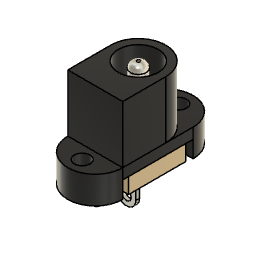
Con_DC-13B_PJ-038BH (Autodesk Fusion 360 design; units mm, degrees)
Autodesk Fusion 360 part; units mm, degrees
note: some values were not read from the file. Set by a fixed rule: which sketch regions a step uses.
sketch "Sketch11" plane through (0, 0, 0) normal (0, 0, 1) x (1, 0, 0)
  circle A0 centre (0, 0) radius 1.25
  circle A1 centre (0, 0) radius 3.2
  line L0 (-10, 0) -> (10, 0) construction
  line L1 (0, 12) -> (0, -25) construction
  line L2 (0, 0) -> (0, -9) construction
  circle A2 centre (0, -9) radius 1.25
  line L3 (0, 0) -> (0, 6.5) construction
  circle A3 centre (0, 6.5) radius 1.25
  line L4 (0, 6.5) -> (0, 9) construction
  line L5 (0, -9) -> (0, -11.5) construction
  line L6 (-4.4, 4.4) -> (-4.4, -6.9)
  line L7 (4.4, 4.4) -> (4.4, -6.9)
  line L8 (-4.4, 9) -> (4.4, 9) construction
  line L9 (-4.4, -11.5) -> (4.4, -11.5) construction
  line L10 (-8, 0) -> (-8, -6.9) construction
  line L11 (-4.4, -6.9) -> (4.4, -6.9)
  arc A4 (-4.4, -6.9) -> (4.4, -6.9) centre (0, -6.9) ccw
  line L12 (0, 6.5) -> (0, 4.4) construction
  line L13 (-4.4, 4.4) -> (4.4, 4.4) construction
  arc A5 (4.4, 4.4) -> (-4.4, 4.4) centre (0, 4.4) ccw
  arc A6 (-1.2373, 0.1776) -> (1.2373, 0.1776) centre (0, 4.4) ccw
  arc A7 (4.4, 0) -> (-4.4, 0) centre (0, 0) ccw
  dimension "d103" = 2.5
  dimension "d104" = 6.4
  dimension "d105" = 9
  dimension "d106" = 2.5
  dimension "d107" = 6.5
  dimension "d108" = 2.5
  dimension "d112" = 2.5
  dimension "d113" = 2.5
  dimension "d114" = 20.5
  dimension "d115" = 4.4
  dimension "d117" = 6.9
  dimension "d118" = 2.1
  dimension "d119" = 2.1
  constraint coincident A0.centre A1.centre
  constraint concentric A0 A1
  constraint horizontal L0
  constraint perpendicular L0 L1
  constraint perpendicular L0 L2
  constraint coincident L2.end A2.centre
  constraint perpendicular L0 L3
  constraint coincident L3.end A3.centre
  constraint parallel L1 L4
  constraint parallel L1 L5
  constraint perpendicular L0 L6
  constraint perpendicular L7 L8
  constraint perpendicular L7 L9
  constraint coincident L0 L10.start
  constraint perpendicular L0 L10
  constraint perpendicular L7 L11
  constraint parallel L1 L12
  constraint perpendicular L7 L13
  constraint coincident A0 A6.end
  constraint coincident A0 A6.start
  constraint concentric A5 A6
  constraint coincident L12.end A7
  constraint tangent L13 A7
  constraint coincident L0 A7.end
  constraint coincident L0 A7.start
  measures "d103" diameter of A0
  measures "d104" diameter of A1
  measures "d105" distance of A0.centre L2.end
  measures "d106" diameter of A2
  measures "d107" distance of A0.centre L3.end
  measures "d108" diameter of A3
  measures "d112" distance of L3.end L4.end
  measures "d113" distance of L2.end L5.end
  measures "d114" distance of L8.start L9.start
  measures "d115" distance of L3 L6
  measures "d117" distance of L10.start L10.end
  measures "d118" distance of L2.end A4.centre
  measures "d119" distance of L3.end L12.end
extrude "Extrude16" add sketch "Sketch11" along normal blind 9.2 contours L6 L7 L11 A7 makes body 1
extrude "Extrude17" add sketch "Sketch11" against normal blind 4.4 separate body contours A0 A6 | A0 A6 | A1 | L6 L7 A5 A7 | L6 L7 L11 A7 | L11 A4 makes body 2
extrude "Extrude18" add sketch "Sketch11" along normal blind 9.2 separate body contours A0 A6 | A0 A6 makes body 3
fillet "Fillet17" radius 1 1 edges at (-1.1654, -0.452, 9.2) on bodies 3
sketch "Sketch12" plane through (4.4, 0, 0) normal (1, 0, 0) x (0, 1, 0)
  line L0 (4.4, 0) -> (-6.9, 0)
  line L1 (-6.9, 0) -> (-6.9, -4.4)
  line L2 (-6.9, -4.4) -> (4.4, -4.4)
  line L3 (4.4, -4.4) -> (4.4, 0)
  line L4 (-6.9, -4.4) -> (4.4, -4.4) construction
  line L5 (4.4, -4.4) -> (4.4, -1.7) construction
  line L6 (4.4, -1.7) -> (-6.9, -1.7)
  line L7 (-6.9, -1.7) -> (-6.9, -4.4) construction
  dimension "d128" = 2.7
  constraint horizontal L4
  constraint vertical L5
  constraint horizontal L6
  constraint vertical L7
  constraint coincident L3 L5.end
  constraint coincident L1.end L2.start
  measures "d128" distance of L1.end L6.end
extrude "Extrude19" cut sketch "Sketch12" against normal blind 8.8 contours L1 L2 L3 L6 bodies 2
sketch "Sketch13" plane through (0, 0, -1.7) normal (0, 0, -1) x (1, 0, 0)
  line L0 (4.4, -4.4) -> (4.4, 6.9)
  line L1 (4.4, 6.9) -> (-4.4, 6.9)
  line L2 (-4.4, 6.9) -> (-4.4, -4.4)
  line L3 (-4.4, -4.4) -> (4.4, -4.4)
  line L4 (4.4, -3.225) -> (-4.4, -3.225)
  line L5 (-4.4, -3.225) -> (-4.4, 5.9743)
  line L6 (-4.4, 5.9743) -> (4.4, 5.9743)
  line L7 (4.4, 5.9743) -> (4.4, -3.225)
  constraint perpendicular L4 L5
  constraint parallel L4 L6
  constraint parallel L5 L7
  constraint coincident L2 L4.end
  constraint perpendicular L2 L4
  constraint coincident L0 L4.start
extrude "Extrude20" add sketch "Sketch13" along normal blind 2.5 separate body contours L0 L2 L4 L5 L6 L7 makes body 4
sketch "Sketch14" plane through (0, 0, -4.2) normal (0, 0, -1) x (1, 0, 0)
  line L0 (4.4, 5.9743) -> (-4.4, 5.9743)
  line L1 (-4.4, 5.9743) -> (-4.4, -3.225)
  line L2 (-4.4, -3.225) -> (4.4, -3.225)
  line L3 (4.4, -3.225) -> (4.4, 5.9743)
  line L4 (0, -5) -> (0, 12) construction
  line L5 (8, 0) -> (-9, 0) construction
  line L6 (-1.4, -4.5489) -> (-1.4, 6) construction
  line L7 (7.8832, 3) -> (-7, 3) construction
  line L8 (8, 5.8) -> (-11, 5.8) construction
  line L9 (-4.9, -5) -> (-4.9, 8) construction
  line L10 (-5.2, -1.5) -> (-4.6, -1.5)
  line L11 (-4.6, -1.5) -> (-4.6, 1.5)
  line L12 (-4.6, 1.5) -> (-5.2, 1.5)
  line L13 (-5.2, 1.5) -> (-5.2, -1.5)
  line L14 (-5.2, -1.5) -> (-4.6, 1.5) construction
  line L15 (-4.6, -1.5) -> (-5.2, 1.5) construction
  line L16 (1.4, -4.5489) -> (1.4, 6) construction
  line L17 (2.9, 2.7) -> (-0.1, 2.7)
  line L18 (-0.1, 2.7) -> (-0.1, 3.3)
  line L19 (-0.1, 3.3) -> (2.9, 3.3)
  line L20 (2.9, 3.3) -> (2.9, 2.7)
  line L21 (-2.9, 5.5) -> (0.1, 5.5)
  line L22 (0.1, 5.5) -> (0.1, 6.1)
  line L23 (0.1, 6.1) -> (-2.9, 6.1)
  line L24 (-2.9, 6.1) -> (-2.9, 5.5)
  line L25 (-2.9, 5.5) -> (0.1, 6.1) construction
  line L26 (0.1, 5.5) -> (-2.9, 6.1) construction
  point P0 (-4.9, 0)
  point P1 (-1.4, 5.8)
  dimension "d136" = 1.4
  dimension "d137" = 3
  dimension "d141" = 5.8
  dimension "d166" = 0.6
  dimension "d167" = 3
  dimension "d177" = 2.8
  dimension "d178" = 3
  dimension "d179" = 0.6
  dimension "d180" = 3
  dimension "d181" = 0.6
  constraint perpendicular L0 L4
  constraint perpendicular L1 L5
  constraint perpendicular L5 L6
  constraint horizontal L10
  constraint perpendicular L10 L11
  constraint parallel L10 L12
  constraint parallel L11 L13
  constraint coincident L14 P0
  constraint coincident L15 P0
  constraint coincident L9 P0
  constraint coincident L5 P0
  constraint horizontal L19
  constraint perpendicular L19 L20
  constraint parallel L17 L19
  constraint parallel L18 L20
  constraint horizontal L21
  constraint perpendicular L21 L22
  constraint parallel L21 L23
  constraint parallel L22 L24
  constraint coincident L25 P1
  constraint coincident L26 P1
  constraint coincident L8 P1
  constraint coincident L6 P1
  measures "d136" distance of L4 L6
  measures "d137" distance of L5 L7
  measures "d141" distance of L5 L8
  measures "d166" distance of L11.end L12.end
  measures "d167" distance of L10.end L11.end
  measures "d178" distance of L17.start L17.end
  measures "d179" distance of L17.start L19.end
  measures "d180" distance of L22.end L23.end
  measures "d181" distance of L21.end L22.end
extrude "Extrude21" add sketch "Sketch14" along normal blind 4.4 separate body contours L0 L21 L22 L24 | L10 L11 L12 L13 | L17 L18 L19 L20 makes body 5 at (-1.9, -5.5, -5.6667) makes body 6 at (-5.2, -0.5, -5.6667) makes body 7 at (1.9, -2.7, -5.6667)
fillet "Fillet18" radius 1.5 6 edges at (-2.9, -5.7371, -8.6) (0.1, -5.7371, -8.6) (-4.9, -1.5, -8.6) (-4.9, 1.5, -8.6) (-0.1, -3, -8.6) (2.9, -3, -8.6) on bodies 5 6 7
sketch "Sketch19" plane through (-4.6, 0, 0) normal (1, 0, 0) x (0, 1, 0)
  arc A0 (-1.5, -7.1) -> (1.5, -7.1) centre (0, -7.1) ccw
  line L0 (1.5, -7.1) -> (1.5, -4.2)
  line L1 (1.5, -4.2) -> (-1.5, -4.2)
  line L2 (-1.5, -4.2) -> (-1.5, -7.1)
  circle A1 centre (0, -7.1) radius 0.75
  dimension "d168" = 1.5
  constraint concentric A0 A1
  measures "d168" diameter of A1
extrude "Extrude23" cut sketch "Sketch19" against normal blind 0.6 contours A1 bodies 6
sketch "Sketch21" plane through (0, -3.3, 0) normal (0, -1, 0) x (1, 0, 0)
  arc A0 (-0.1, -7.1) -> (2.9, -7.1) centre (1.4, -7.1) ccw
  line L0 (2.9, -7.1) -> (2.9, -4.2)
  line L1 (2.9, -4.2) -> (-0.1, -4.2)
  line L2 (-0.1, -4.2) -> (-0.1, -7.1)
  circle A1 centre (1.4, -7.1) radius 0.75
  dimension "d182" = 1.5
  constraint concentric A0 A1
  measures "d182" diameter of A1
extrude "Extrude29" cut sketch "Sketch21" against normal blind 0.6 contours A1 bodies 7
sketch "Sketch22" plane through (0, -5.9743, 0) normal (0, -1, 0) x (1, 0, 0)
  arc A0 (-2.9, -7.1) -> (0.1, -7.1) centre (-1.4, -7.1) ccw
  line L0 (0.1, -7.1) -> (0.1, -4.2)
  line L1 (0.1, -4.2) -> (-2.9, -4.2)
  line L2 (-2.9, -4.2) -> (-2.9, -7.1)
  circle A1 centre (-1.4, -7.1) radius 0.75
  dimension "d185" = 1.5
  constraint concentric A0 A1
  measures "d185" diameter of A1
extrude "Extrude30" cut sketch "Sketch22" against normal blind 0.6 contours A1 bodies 5
sketch "Sketch20" plane through (-4.6, 0, 0) normal (1, 0, 0) x (0, 1, 0)
  arc A0 (-1.5, -7.1) -> (1.5, -7.1) centre (0, -7.1) ccw
  line L0 (1.5, -7.1) -> (1.5, -4.2)
  line L1 (1.5, -4.2) -> (-1.5, -4.2)
  line L2 (-1.5, -4.2) -> (-1.5, -7.1)
  line L3 (1.5, -4.2) -> (-1.5, -4.2)
  line L4 (-1.5, -4.2) -> (-1.5, -4.8)
  line L5 (-1.5, -4.8) -> (1.5, -4.8)
  line L6 (1.5, -4.8) -> (1.5, -4.2)
  circle A1 centre (0, -7.1) radius 0.75
  dimension "d171" = 3
  dimension "d172" = 0.6
  constraint horizontal L3
  constraint vertical L4
  constraint horizontal L5
  constraint vertical L6
  constraint coincident L0.end L1.start
  measures "d171" distance of L0.end L1.end
  measures "d172" distance of L0.end L5.end
extrude "Extrude28" add sketch "Sketch20" along normal blind 6.5 separate body contours L0 L1 L2 L3 L4 L5 L6 makes body 8
extrude "Extrude26" cut sketch "Sketch11" against normal blind 2.7 contours A0 A6 | A0 A6 bodies 2 4
fillet "Fillet20" radius 0.8 2 edges at (1.9, -1.5, -4.5) (1.9, 1.5, -4.5) on bodies 8
